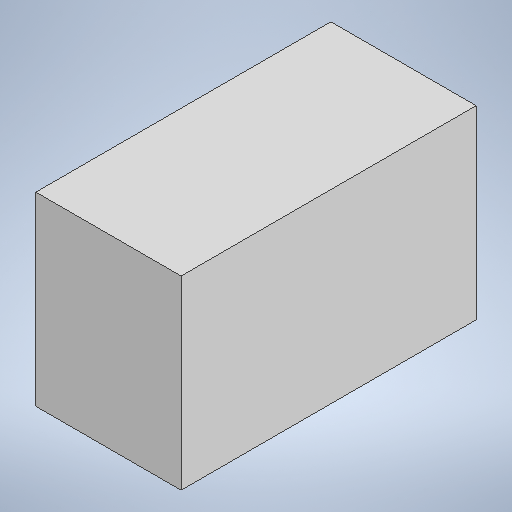
# Autodesk Inventor part: Outer Case
Saved by Autodesk Inventor 2025.2 (Build 292293000, 293)
## iProperties
Created: 2024-12-06
Part Number: Outer Case
Material: Generic
Document SubType Name: Modeling
Designer: cbast
Density: 1 g/cm^3
Appearance: Default
Author: cbast
Autodesk Inventor part; units mm, degrees
ref_plane "YZ Plane" through (0, 0, 0) normal (1, 0, 0) x (0, 1, 0)
ref_plane "XZ Plane" through (0, 0, 0) normal (0, 1, 0) x (-1, 0, 0)
ref_plane "XY Plane" through (0, 0, 0) normal (0, 0, 1) x (1, 0, 0)
sketch "Sketch1" plane through (0, 0, 0) normal (0, 1, 0) x (-1, 0, 0)
  line L0 (27.5, 61) -> (-27.5, 61)
  line L1 (-27.5, 61) -> (-27.5, -61)
  line L2 (-27.5, -61) -> (27.5, -61)
  line L3 (27.5, -61) -> (27.5, 61)
  line L4 (27.5, 61) -> (-27.5, -61) construction
  line L5 (-27.5, 61) -> (27.5, -61) construction
  line L6 (32.5, 66) -> (-32.5, 66)
  line L7 (-32.5, 66) -> (-32.5, -66)
  line L8 (-32.5, -66) -> (32.5, -66)
  line L9 (32.5, -66) -> (32.5, 66)
  line L10 (32.5, 66) -> (-32.5, -66) construction
  line L11 (-32.5, 66) -> (32.5, -66) construction
  point P0 (0, 0)
  dimension "d0" = 122
  dimension "d1" = 55
  dimension "d10" = 5
  dimension "d11" = 5
  constraints: 24 end point, 4 midpoint, 4 parallel, 2 horizontal, 2 perpendicular
  measures "d0" distance of L2.end L0.start
  measures "d1" distance of L1.end L2.end
  measures "d10" distance between parallel lines of L9 L3
  measures "d11" distance between parallel lines of L8 L2
extrude "Extrusion1" add sketch "Sketch1" along normal blind 78
sketch "Sketch5" plane through (0, 78, 0) normal (0, 1, 0) x (1, 0, 0)
  line L0 (32.5, 66) -> (-32.5, 66)
  line L1 (-32.5, 66) -> (-32.5, -66)
  line L2 (-32.5, -66) -> (32.5, -66)
  line L3 (32.5, -66) -> (32.5, 66)
  line L4 (32.5, 66) -> (-32.5, -66) construction
  line L5 (-32.5, 66) -> (32.5, -66) construction
  point P0 (0, 0)
  dimension "d20" = 65
  dimension "d21" = 132
  constraints: 12 end point, 2 midpoint, 2 parallel, 1 horizontal, 1 perpendicular
  measures "d20" distance of L2.end L1.end
  measures "d21" distance of L1.end L0.end
extrude "Extrusion5" add sketch "Sketch5" along normal blind 5
body "Solid1"
